Autodesk Fusion 360 part; units mm, degrees
note: some values were not read from the file. Set by a fixed rule: which sketch regions a step uses.
(part 10 of 20)
  spline S55 degree 5 poles (-13.208, 9.0304) (-13.2069, 9.0286) (-13.2047, 9.0249) (-13.2015, 9.0195) (-13.1971, 9.0122) (-13.1916, 9.0031) (-13.1862, 8.9941) (-13.1807, 8.9851) (-13.1752, 8.9761) (-13.1698, 8.9671) (-13.1643, 8.9582) (-13.1589, 8.9493) (-13.1534, 8.9405) (-13.1479, 8.9317) (-13.1425, 8.9229) (-13.137, 8.9141) (-13.1315, 8.9054) (-13.1261, 8.8967) (-13.1206, 8.888) (-13.1151, 8.8794) (-13.1097, 8.8708) (-13.1042, 8.8622) (-13.0988, 8.8537) (-13.0933, 8.8452) (-13.0878, 8.8367) (-13.0824, 8.8283) (-13.0769, 8.8199) (-13.0715, 8.8115) (-13.066, 8.8032) (-13.0606, 8.7948) (-13.0551, 8.7866) (-13.0497, 8.7783) (-13.0442, 8.7701) (-13.0388, 8.7619) (-13.0333, 8.7538) (-13.0279, 8.7456) (-13.0224, 8.7376) (-13.017, 8.7295) (-13.0116, 8.7215) (-13.0062, 8.7135) (-13.0007, 8.7055) (-12.9953, 8.6976) (-12.9899, 8.6897) (-12.9845, 8.6819) (-12.9791, 8.6741) (-12.9736, 8.6663) (-12.9682, 8.6585) (-12.9628, 8.6508) (-12.9574, 8.6431) (-12.9521, 8.6354) (-12.9467, 8.6278) (-12.9413, 8.6202) (-12.9359, 8.6126) (-12.9305, 8.6051) (-12.9252, 8.5976) (-12.9198, 8.5902) (-12.9144, 8.5827) (-12.9091, 8.5754) (-12.9037, 8.568) (-12.8984, 8.5607) (-12.893, 8.5534) (-12.8877, 8.5461) (-12.8824, 8.5389) (-12.8771, 8.5317) (-12.8718, 8.5246) (-12.8664, 8.5174) (-12.8611, 8.5103) (-12.8558, 8.5033) (-12.8506, 8.4963) (-12.8453, 8.4893) (-12.84, 8.4823) (-12.8347, 8.4754) (-12.8295, 8.4685) (-12.8242, 8.4617) (-12.819, 8.4549) (-12.8138, 8.4481) (-12.8085, 8.4413) (-12.8033, 8.4346) (-12.7981, 8.4279) (-12.7929, 8.4213) (-12.7877, 8.4147) (-12.7825, 8.4081) (-12.7773, 8.4016) (-12.7722, 8.3951) (-12.767, 8.3886) (-12.7619, 8.3822) (-12.7567, 8.3758) (-12.7516, 8.3694) (-12.7465, 8.3631) (-12.7414, 8.3568) (-12.7363, 8.3505) (-12.7312, 8.3443) (-12.7261, 8.3381) (-12.721, 8.332) (-12.716, 8.3259) (-12.7109, 8.3198) (-12.7059, 8.3137) (-12.7009, 8.3077) (-12.6959, 8.3017) (-12.6909, 8.2958) (-12.6859, 8.2899) (-12.6809, 8.284) (-12.676, 8.2782) (-12.671, 8.2724) (-12.6661, 8.2666) (-12.6612, 8.2609) (-12.6562, 8.2552) (-12.6513, 8.2496) (-12.6465, 8.2439) (-12.6416, 8.2384) (-12.6367, 8.2328) (-12.6319, 8.2273) (-12.6271, 8.2218) (-12.6223, 8.2164) (-12.6175, 8.211) (-12.6127, 8.2056) (-12.6079, 8.2003) (-12.6032, 8.195) (-12.5984, 8.1898) (-12.5937, 8.1846) (-12.589, 8.1794) (-12.5843, 8.1742) (-12.5796, 8.1691) (-12.575, 8.1641) (-12.5703, 8.159) (-12.5657, 8.154) (-12.5611, 8.1491) (-12.5565, 8.1441) (-12.552, 8.1393) (-12.5474, 8.1344) (-12.5429, 8.1296) (-12.5384, 8.1248) (-12.5339, 8.1201) (-12.5294, 8.1154) (-12.5249, 8.1107) (-12.5205, 8.1061) (-12.5161, 8.1015) (-12.5117, 8.097) (-12.5073, 8.0925) (-12.5029, 8.088) (-12.4986, 8.0836) (-12.4943, 8.0792) (-12.49, 8.0748) (-12.4857, 8.0705) (-12.4815, 8.0662) (-12.4772, 8.062) (-12.473, 8.0578) (-12.4688, 8.0536) (-12.4647, 8.0495) (-12.4605, 8.0454) (-12.4564, 8.0413) (-12.4523, 8.0373) (-12.4482, 8.0333) (-12.4442, 8.0294) (-12.4401, 8.0255) (-12.4361, 8.0216) (-12.4322, 8.0178) (-12.4282, 8.014) (-12.4243, 8.0103) (-12.4204, 8.0066) (-12.4165, 8.0029) (-12.4127, 7.9993) (-12.4089, 7.9957) (-12.4051, 7.9922) (-12.4013, 7.9887) (-12.3976, 7.9852) (-12.3938, 7.9818) (-12.3902, 7.9784) (-12.3865, 7.975) (-12.3829, 7.9717) (-12.3793, 7.9684) (-12.3757, 7.9652) (-12.3722, 7.962) (-12.3687, 7.9589) (-12.3652, 7.9558) (-12.3617, 7.9527) (-12.3583, 7.9496) (-12.3549, 7.9467) (-12.3516, 7.9437) (-12.3483, 7.9408) (-12.345, 7.9379) (-12.3417, 7.9351) (-12.3385, 7.9323) (-12.3353, 7.9296) (-12.3322, 7.9268) (-12.329, 7.9242) (-12.326, 7.9216) (-12.3229, 7.919) (-12.3199, 7.9164) (-12.3169, 7.9139) (-12.314, 7.9115) (-12.3111, 7.909) (-12.3082, 7.9066) (-12.3054, 7.9043) (-12.3026, 7.902) (-12.2998, 7.8998) (-12.2971, 7.8975) (-12.2944, 7.8954) (-12.2918, 7.8932) (-12.2892, 7.8911) (-12.2867, 7.8891) (-12.2841, 7.8871) (-12.2817, 7.8851) (-12.2792, 7.8832) (-12.2769, 7.8813) (-12.2745, 7.8795) (-12.2722, 7.8777) (-12.27, 7.8759) (-12.2677, 7.8742) (-12.2656, 7.8726) (-12.2635, 7.8709) (-12.2614, 7.8693) (-12.2594, 7.8678) (-12.2574, 7.8663) (-12.2555, 7.8649) (-12.2536, 7.8634) (-12.2517, 7.8621) (-12.25, 7.8608) (-12.2482, 7.8595) (-12.2465, 7.8582) (-12.2449, 7.857) (-12.2433, 7.8559) (-12.2418, 7.8548) (-12.2403, 7.8537) (-12.2389, 7.8527) (-12.2376, 7.8517) (-12.2363, 7.8508) (-12.235, 7.8499) (-12.2338, 7.8491) (-12.2327, 7.8483) (-12.2316, 7.8475) (-12.2306, 7.8468) (-12.2296, 7.8462) (-12.2287, 7.8455) (-12.2279, 7.845) (-12.2271, 7.8445) (-12.2264, 7.844) (-12.2258, 7.8435) (-12.2252, 7.8431) (-12.2247, 7.8428) (-12.2242, 7.8425) (-12.2239, 7.8423) (-12.2237, 7.8422) (-12.2236, 7.8421) (-12.2236, 7.8421) knots -1 -1 -1 -1 -1 -1 -0.99583333 -0.99166667 -0.9875 -0.98333333 -0.97916667 -0.975 -0.97083333 -0.96666667 -0.9625 -0.95833333 -0.95416667 -0.95 -0.94583333 -0.94166667 -0.9375 -0.93333333 -0.92916667 -0.925 -0.92083333 -0.91666667 -0.9125 -0.90833333 -0.90416667 -0.9 -0.89583333 -0.89166667 -0.8875 -0.88333333 -0.87916667 -0.875 -0.87083333 -0.86666667 -0.8625 -0.85833333 -0.85416667 -0.85 -0.84583333 -0.84166667 -0.8375 -0.83333333 -0.82916667 -0.825 -0.82083333 -0.81666667 -0.8125 -0.80833333 -0.80416667 -0.8 -0.79583333 -0.79166667 -0.7875 -0.78333333 -0.77916667 -0.775 -0.77083333 -0.76666667 -0.7625 -0.75833333 -0.75416667 -0.75 -0.74583333 -0.74166667 -0.7375 -0.73333333 -0.72916667 -0.725 -0.72083333 -0.71666667 -0.7125 -0.70833333 -0.70416667 -0.7 -0.69583333 -0.69166667 -0.6875 -0.68333333 -0.67916667 -0.675 -0.67083333 -0.66666667 -0.6625 -0.65833333 -0.65416667 -0.65 -0.64583333 -0.64166667 -0.6375 -0.63333333 -0.62916667 -0.625 -0.62083333 -0.61666667 -0.6125 -0.60833333 -0.60416667 -0.6 -0.59583333 -0.59166667 -0.5875 -0.58333333 -0.57916667 -0.575 -0.57083333 -0.56666667 -0.5625 -0.55833333 -0.55416667 -0.55 -0.54583333 -0.54166667 -0.5375 -0.53333333 -0.52916667 -0.525 -0.52083333 -0.51666667 -0.5125 -0.50833333 -0.50416667 -0.5 -0.49583333 -0.49166667 -0.4875 -0.48333333 -0.47916667 -0.475 -0.47083333 -0.46666667 -0.4625 -0.45833333 -0.45416667 -0.45 -0.44583333 -0.44166667 -0.4375 -0.43333333 -0.42916667 -0.425 -0.42083333 -0.41666667 -0.4125 -0.40833333 -0.40416667 -0.4 -0.39583333 -0.39166667 -0.3875 -0.38333333 -0.37916667 -0.375 -0.37083333 -0.36666667 -0.3625 -0.35833333 -0.35416667 -0.35 -0.34583333 -0.34166667 -0.3375 -0.33333333 -0.32916667 -0.325 -0.32083333 -0.31666667 -0.3125 -0.30833333 -0.30416667 -0.3 -0.29583333 -0.29166667 -0.2875 -0.28333333 -0.27916667 -0.275 -0.27083333 -0.26666667 -0.2625 -0.25833333 -0.25416667 -0.25 -0.24583333 -0.24166667 -0.2375 -0.23333333 -0.22916667 -0.225 -0.22083333 -0.21666667 -0.2125 -0.20833333 -0.20416667 -0.2 -0.19583333 -0.19166667 -0.1875 -0.18333333 -0.17916667 -0.175 -0.17083333 -0.16666667 -0.1625 -0.15833333 -0.15416667 -0.15 -0.14583333 -0.14166667 -0.1375 -0.13333333 -0.12916667 -0.125 -0.12083333 -0.11666667 -0.1125 -0.10833333 -0.10416667 -0.1 -0.09583333 -0.09166667 -0.0875 -0.08333333 -0.07916667 -0.075 -0.07083333 -0.06666667 -0.0625 -0.05833333 -0.05416667 -0.05 -0.04583333 -0.04166667 -0.0375 -0.03333333 -0.02916667 -0.025 -0.02083333 -0.01666667 -0.0125 -0.00833333 -0.00416667 0 0 0 0 0 0
  line L110 (-12.2236, 7.8421) -> (-12.223, 7.8417)
  line L111 (-12.223, 7.8417) -> (-11.5731, 7.4247)
  arc A56 (-11.5731, 7.4247) -> (-12.2165, 6.3102) centre (0, 0) ccw
  line L112 (-12.2165, 6.3102) -> (-12.9026, 6.6646)
  line L113 (-12.9026, 6.6646) -> (-12.9032, 6.6649)
  spline S56 degree 5 poles (-12.9032, 6.6649) (-12.9033, 6.6649) (-12.9034, 6.665) (-12.9036, 6.6651) (-12.9039, 6.6652) (-12.9044, 6.6655) (-12.905, 6.6658) (-12.9056, 6.6661) (-12.9063, 6.6664) (-12.9071, 6.6668) (-12.9079, 6.6672) (-12.9088, 6.6676) (-12.9098, 6.6681) (-12.9108, 6.6686) (-12.912, 6.6691) (-12.9132, 6.6697) (-12.9144, 6.6703) (-12.9157, 6.6709) (-12.9171, 6.6715) (-12.9186, 6.6722) (-12.9201, 6.6729) (-12.9217, 6.6736) (-12.9234, 6.6743) (-12.9251, 6.6751) (-12.9269, 6.6759) (-12.9287, 6.6767) (-12.9306, 6.6775) (-12.9326, 6.6784) (-12.9346, 6.6793) (-12.9367, 6.6802) (-12.9389, 6.6811) (-12.9411, 6.6821) (-12.9434, 6.683) (-12.9457, 6.684) (-12.9482, 6.685) (-12.9506, 6.686) (-12.9531, 6.6871) (-12.9557, 6.6881) (-12.9584, 6.6892) (-12.9611, 6.6903) (-12.9638, 6.6914) (-12.9667, 6.6925) (-12.9695, 6.6937) (-12.9725, 6.6948) (-12.9755, 6.696) (-12.9785, 6.6972) (-12.9816, 6.6984) (-12.9848, 6.6996) (-12.988, 6.7008) (-12.9913, 6.7021) (-12.9946, 6.7033) (-12.998, 6.7046) (-13.0015, 6.7059) (-13.005, 6.7072) (-13.0085, 6.7085) (-13.0121, 6.7098) (-13.0158, 6.7111) (-13.0195, 6.7125) (-13.0232, 6.7138) (-13.0271, 6.7152) (-13.0309, 6.7165) (-13.0349, 6.7179) (-13.0388, 6.7193) (-13.0429, 6.7207) (-13.0469, 6.7221) (-13.0511, 6.7235) (-13.0552, 6.7249) (-13.0595, 6.7264) (-13.0638, 6.7278) (-13.0681, 6.7292) (-13.0725, 6.7307) (-13.0769, 6.7321) (-13.0814, 6.7336) (-13.0859, 6.7351) (-13.0905, 6.7366) (-13.0951, 6.738) (-13.0998, 6.7395) (-13.1046, 6.741) (-13.1093, 6.7425) (-13.1142, 6.744) (-13.119, 6.7455) (-13.124, 6.747) (-13.1289, 6.7485) (-13.1339, 6.75) (-13.139, 6.7516) (-13.1441, 6.7531) (-13.1493, 6.7546) (-13.1545, 6.7561) (-13.1597, 6.7577) (-13.165, 6.7592) (-13.1704, 6.7607) (-13.1758, 6.7623) (-13.1812, 6.7638) (-13.1867, 6.7653) (-13.1922, 6.7669) (-13.1978, 6.7684) (-13.2034, 6.77) (-13.209, 6.7715) (-13.2147, 6.7731) (-13.2205, 6.7746) (-13.2263, 6.7761) (-13.2321, 6.7777) (-13.238, 6.7792) (-13.2439, 6.7808) (-13.2499, 6.7823) (-13.2559, 6.7839) (-13.2619, 6.7854) (-13.268, 6.7869) (-13.2742, 6.7885) (-13.2804, 6.79) (-13.2866, 6.7915) (-13.2928, 6.7931) (-13.2991, 6.7946) (-13.3055, 6.7961) (-13.3119, 6.7976) (-13.3183, 6.7992) (-13.3248, 6.8007) (-13.3313, 6.8022) (-13.3379, 6.8037) (-13.3445, 6.8052) (-13.3511, 6.8067) (-13.3578, 6.8082) (-13.3645, 6.8097) (-13.3712, 6.8112) (-13.378, 6.8127) (-13.3849, 6.8142) (-13.3918, 6.8157) (-13.3987, 6.8171) (-13.4056, 6.8186) (-13.4126, 6.8201) (-13.4197, 6.8215) (-13.4267, 6.823) (-13.4339, 6.8244) (-13.441, 6.8259) (-13.4482, 6.8273) (-13.4554, 6.8288) (-13.4627, 6.8302) (-13.47, 6.8316) (-13.4773, 6.833) (-13.4847, 6.8344) (-13.4922, 6.8358) (-13.4996, 6.8372) (-13.5071, 6.8386) (-13.5146, 6.84) (-13.5222, 6.8414) (-13.5298, 6.8427) (-13.5375, 6.8441) (-13.5451, 6.8454) (-13.5528, 6.8468) (-13.5606, 6.8481) (-13.5684, 6.8494) (-13.5762, 6.8508) (-13.5841, 6.8521) (-13.592, 6.8534) (-13.5999, 6.8547) (-13.6079, 6.856) (-13.6159, 6.8572) (-13.6239, 6.8585) (-13.632, 6.8598) (-13.6401, 6.861) (-13.6483, 6.8623) (-13.6564, 6.8635) (-13.6647, 6.8647) (-13.6729, 6.8659) (-13.6812, 6.8671) (-13.6895, 6.8683) (-13.6979, 6.8695) (-13.7063, 6.8707) (-13.7147, 6.8718) (-13.7231, 6.873) (-13.7316, 6.8741) (-13.7401, 6.8753) (-13.7487, 6.8764) (-13.7573, 6.8775) (-13.7659, 6.8786) (-13.7746, 6.8797) (-13.7833, 6.8808) (-13.792, 6.8818) (-13.8007, 6.8829) (-13.8095, 6.884) (-13.8184, 6.885) (-13.8272, 6.886) (-13.8361, 6.887) (-13.845, 6.888) (-13.854, 6.889) (-13.8629, 6.89) (-13.872, 6.891) (-13.881, 6.8919) (-13.8901, 6.8929) (-13.8992, 6.8938) (-13.9083, 6.8947) (-13.9175, 6.8956) (-13.9267, 6.8965) (-13.936, 6.8974) (-13.9452, 6.8982) (-13.9545, 6.8991) (-13.9639, 6.8999) (-13.9732, 6.9008) (-13.9826, 6.9016) (-13.992, 6.9024) (-14.0015, 6.9032) (-14.011, 6.9039) (-14.0205, 6.9047) (-14.03, 6.9055) (-14.0396, 6.9062) (-14.0492, 6.9069) (-14.0588, 6.9076) (-14.0685, 6.9083) (-14.0782, 6.909) (-14.0879, 6.9097) (-14.0976, 6.9103) (-14.1074, 6.9109) (-14.1172, 6.9116) (-14.1271, 6.9122) (-14.1369, 6.9128) (-14.1468, 6.9134) (-14.1568, 6.9139) (-14.1667, 6.9145) (-14.1767, 6.915) (-14.1867, 6.9155) (-14.1967, 6.916) (-14.2068, 6.9165) (-14.2169, 6.917) (-14.227, 6.9175) (-14.2372, 6.9179) (-14.2474, 6.9183) (-14.2576, 6.9188) (-14.2678, 6.9192) (-14.2781, 6.9195) (-14.2883, 6.9199) (-14.2987, 6.9203) (-14.309, 6.9206) (-14.3194, 6.9209) (-14.3298, 6.9212) (-14.3402, 6.9215) (-14.3507, 6.9218) (-14.3611, 6.9221) (-14.3716, 6.9223) (-14.3822, 6.9225) (-14.3927, 6.9227) (-14.4033, 6.9229) (-14.4118, 6.9231) (-14.4182, 6.9232) (-14.4224, 6.9232) (-14.4246, 6.9233) knots 0 0 0 0 0 0 0.00416667 0.00833333 0.0125 0.01666667 0.02083333 0.025 0.02916667 0.03333333 0.0375 0.04166667 0.04583333 0.05 0.05416667 0.05833333 0.0625 0.06666667 0.07083333 0.075 0.07916667 0.08333333 0.0875 0.09166667 0.09583333 0.1 0.10416667 0.10833333 0.1125 0.11666667 0.12083333 0.125 0.12916667 0.13333333 0.1375 0.14166667 0.14583333 0.15 0.15416667 0.15833333 0.1625 0.16666667 0.17083333 0.175 0.17916667 0.18333333 0.1875 0.19166667 0.19583333 0.2 0.20416667 0.20833333 0.2125 0.21666667 0.22083333 0.225 0.22916667 0.23333333 0.2375 0.24166667 0.24583333 0.25 0.25416667 0.25833333 0.2625 0.26666667 0.27083333 0.275 0.27916667 0.28333333 0.2875 0.29166667 0.29583333 0.3 0.30416667 0.30833333 0.3125 0.31666667 0.32083333 0.325 0.32916667 0.33333333 0.3375 0.34166667 0.34583333 0.35 0.35416667 0.35833333 0.3625 0.36666667 0.37083333 0.375 0.37916667 0.38333333 0.3875 0.39166667 0.39583333 0.4 0.40416667 0.40833333 0.4125 0.41666667 0.42083333 0.425 0.42916667 0.43333333 0.4375 0.44166667 0.44583333 0.45 0.45416667 0.45833333 0.4625 0.46666667 0.47083333 0.475 0.47916667 0.48333333 0.4875 0.49166667 0.49583333 0.5 0.50416667 0.50833333 0.5125 0.51666667 0.52083333 0.525 0.52916667 0.53333333 0.5375 0.54166667 0.54583333 0.55 0.55416667 0.55833333 0.5625 0.56666667 0.57083333 0.575 0.57916667 0.58333333 0.5875 0.59166667 0.59583333 0.6 0.60416667 0.60833333 0.6125 0.61666667 0.62083333 0.625 0.62916667 0.63333333 0.6375 0.64166667 0.64583333 0.65 0.65416667 0.65833333 0.6625 0.66666667 0.67083333 0.675 0.67916667 0.68333333 0.6875 0.69166667 0.69583333 0.7 0.70416667 0.70833333 0.7125 0.71666667 0.72083333 0.725 0.72916667 0.73333333 0.7375 0.74166667 0.74583333 0.75 0.75416667 0.75833333 0.7625 0.76666667 0.77083333 0.775 0.77916667 0.78333333 0.7875 0.79166667 0.79583333 0.8 0.80416667 0.80833333 0.8125 0.81666667 0.82083333 0.825 0.82916667 0.83333333 0.8375 0.84166667 0.84583333 0.85 0.85416667 0.85833333 0.8625 0.86666667 0.87083333 0.875 0.87916667 0.88333333 0.8875 0.89166667 0.89583333 0.9 0.90416667 0.90833333 0.9125 0.91666667 0.92083333 0.925 0.92916667 0.93333333 0.9375 0.94166667 0.94583333 0.95 0.95416667 0.95833333 0.9625 0.96666667 0.97083333 0.975 0.97916667 0.98333333 0.9875 0.99166667 0.99583333 1 1 1 1 1 1
  arc A57 (-14.4246, 6.9233) -> (-14.7969, 6.087) centre (0, 0) ccw
  spline S57 degree 5 poles (-14.7969, 6.087) (-14.7955, 6.0854) (-14.7926, 6.0823) (-14.7882, 6.0776) (-14.7824, 6.0714) (-14.7752, 6.0637) (-14.768, 6.056) (-14.7608, 6.0483) (-14.7536, 6.0406) (-14.7464, 6.033) (-14.7392, 6.0254) (-14.732, 6.0179) (-14.7248, 6.0104) (-14.7176, 6.0029) (-14.7104, 5.9954) (-14.7033, 5.988) (-14.6961, 5.9806) (-14.689, 5.9732) (-14.6818, 5.9659) (-14.6747, 5.9586) (-14.6675, 5.9513) (-14.6604, 5.9441) (-14.6533, 5.9368) (-14.6462, 5.9297) (-14.6391, 5.9225) (-14.632, 5.9154) (-14.6249, 5.9083) (-14.6178, 5.9012) (-14.6108, 5.8942) (-14.6037, 5.8872) (-14.5966, 5.8802) (-14.5896, 5.8733) (-14.5826, 5.8664) (-14.5755, 5.8595) (-14.5685, 5.8527) (-14.5615, 5.8459) (-14.5545, 5.8391) (-14.5475, 5.8324) (-14.5405, 5.8256) (-14.5336, 5.819) (-14.5266, 5.8123) (-14.5197, 5.8057) (-14.5127, 5.7991) (-14.5058, 5.7925) (-14.4989, 5.786) (-14.492, 5.7795) (-14.4851, 5.773) (-14.4782, 5.7666) (-14.4713, 5.7602) (-14.4644, 5.7538) (-14.4576, 5.7475) (-14.4507, 5.7412) (-14.4439, 5.7349) (-14.4371, 5.7287) (-14.4303, 5.7225) (-14.4235, 5.7163) (-14.4167, 5.7101) (-14.4099, 5.704) (-14.4031, 5.6979) (-14.3964, 5.6919) (-14.3896, 5.6859) (-14.3829, 5.6799) (-14.3762, 5.6739) (-14.3695, 5.668) (-14.3628, 5.6621) (-14.3562, 5.6562) (-14.3495, 5.6504) (-14.3429, 5.6446) (-14.3362, 5.6388) (-14.3296, 5.6331) (-14.323, 5.6274) (-14.3164, 5.6217) (-14.3098, 5.6161) (-14.3033, 5.6105) (-14.2967, 5.6049) (-14.2902, 5.5993) (-14.2837, 5.5938) (-14.2772, 5.5883) (-14.2707, 5.5829) (-14.2642, 5.5775) (-14.2578, 5.5721) (-14.2513, 5.5667) (-14.2449, 5.5614) (-14.2385, 5.5561) (-14.2321, 5.5509) (-14.2257, 5.5457) (-14.2194, 5.5405) (-14.213, 5.5353) (-14.2067, 5.5302) (-14.2004, 5.5251) (-14.1941, 5.52) (-14.1879, 5.515) (-14.1816, 5.51) (-14.1754, 5.505) (-14.1692, 5.5001) (-14.163, 5.4952) (-14.1568, 5.4903) (-14.1506, 5.4855) (-14.1445, 5.4807) (-14.1383, 5.4759) (-14.1322, 5.4712) (-14.1262, 5.4665) (-14.1201, 5.4618) (-14.114, 5.4572) (-14.108, 5.4526) (-14.102, 5.448) (-14.096, 5.4434) (-14.0901, 5.4389) (-14.0841, 5.4344) (-14.0782, 5.43) (-14.0723, 5.4256) (-14.0664, 5.4212) (-14.0606, 5.4169) (-14.0547, 5.4125) (-14.0489, 5.4083) (-14.0431, 5.404) (-14.0373, 5.3998) (-14.0316, 5.3956) (-14.0259, 5.3914) (-14.0202, 5.3873) (-14.0145, 5.3832) (-14.0088, 5.3792) (-14.0032, 5.3752) (-13.9976, 5.3712) (-13.992, 5.3672) (-13.9865, 5.3633) (-13.9809, 5.3594) (-13.9754, 5.3555) (-13.9699, 5.3517) (-13.9645, 5.3479) (-13.959, 5.3441) (-13.9536, 5.3404) (-13.9482, 5.3367) (-13.9429, 5.3331) (-13.9376, 5.3294) (-13.9322, 5.3258) (-13.927, 5.3223) (-13.9217, 5.3187) (-13.9165, 5.3152) (-13.9113, 5.3118) (-13.9061, 5.3083) (-13.901, 5.3049) (-13.8959, 5.3015) (-13.8908, 5.2982) (-13.8858, 5.2949) (-13.8807, 5.2916) (-13.8757, 5.2884) (-13.8708, 5.2852) (-13.8658, 5.282) (-13.8609, 5.2789) (-13.8561, 5.2758) (-13.8512, 5.2727) (-13.8464, 5.2697) (-13.8416, 5.2666) (-13.8369, 5.2637) (-13.8322, 5.2607) (-13.8275, 5.2578) (-13.8228, 5.2549) (-13.8182, 5.2521) (-13.8136, 5.2493) (-13.8091, 5.2465) (-13.8046, 5.2438) (-13.8001, 5.241) (-13.7956, 5.2384) (-13.7912, 5.2357) (-13.7869, 5.2331) (-13.7825, 5.2305) (-13.7782, 5.228) (-13.7739, 5.2254) (-13.7697, 5.223) (-13.7655, 5.2205) (-13.7613, 5.2181) (-13.7572, 5.2157) (-13.7531, 5.2134) (-13.7491, 5.211) (-13.7451, 5.2087) (-13.7411, 5.2065) (-13.7372, 5.2043) (-13.7333, 5.2021) (-13.7294, 5.1999) (-13.7256, 5.1978) (-13.7218, 5.1957) (-13.7181, 5.1936) (-13.7144, 5.1916) (-13.7108, 5.1896) (-13.7072, 5.1877) (-13.7036, 5.1857) (-13.7001, 5.1838) (-13.6966, 5.182) (-13.6932, 5.1801) (-13.6898, 5.1783) (-13.6864, 5.1766) (-13.6831, 5.1749) (-13.6799, 5.1732) (-13.6767, 5.1715) (-13.6735, 5.1698) (-13.6704, 5.1682) (-13.6673, 5.1667) (-13.6643, 5.1651) (-13.6613, 5.1636) (-13.6584, 5.1622) (-13.6555, 5.1607) (-13.6527, 5.1593) (-13.6499, 5.1579) (-13.6472, 5.1566) (-13.6445, 5.1553) (-13.6419, 5.154) (-13.6393, 5.1528) (-13.6368, 5.1515) (-13.6343, 5.1504) (-13.6319, 5.1492) (-13.6296, 5.1481) (-13.6273, 5.147) (-13.625, 5.146) (-13.6228, 5.1449) (-13.6207, 5.1439) (-13.6186, 5.143) (-13.6166, 5.1421) (-13.6147, 5.1412) (-13.6128, 5.1403) (-13.6109, 5.1395) (-13.6091, 5.1387) (-13.6074, 5.1379) (-13.6057, 5.1372) (-13.6042, 5.1365) (-13.6026, 5.1358) (-13.6011, 5.1352) (-13.5997, 5.1346) (-13.5984, 5.134) (-13.5971, 5.1335) (-13.5959, 5.1329) (-13.5948, 5.1325) (-13.5937, 5.132) (-13.5927, 5.1316) (-13.5918, 5.1312) (-13.5909, 5.1309) (-13.5901, 5.1305) (-13.5894, 5.1303) (-13.5887, 5.13) (-13.5882, 5.1298) (-13.5877, 5.1296) (-13.5873, 5.1294) (-13.5871, 5.1293) (-13.587, 5.1293) (-13.5869, 5.1293) knots -1 -1 -1 -1 -1 -1 -0.99583333 -0.99166667 -0.9875 -0.98333333 -0.97916667 -0.975 -0.97083333 -0.96666667 -0.9625 -0.95833333 -0.95416667 -0.95 -0.94583333 -0.94166667 -0.9375 -0.93333333 -0.92916667 -0.925 -0.92083333 -0.91666667 -0.9125 -0.90833333 -0.90416667 -0.9 -0.89583333 -0.89166667 -0.8875 -0.88333333 -0.87916667 -0.875 -0.87083333 -0.86666667 -0.8625 -0.85833333 -0.85416667 -0.85 -0.84583333 -0.84166667 -0.8375 -0.83333333 -0.82916667 -0.825 -0.82083333 -0.81666667 -0.8125 -0.80833333 -0.80416667 -0.8 -0.79583333 -0.79166667 -0.7875 -0.78333333 -0.77916667 -0.775 -0.77083333 -0.76666667 -0.7625 -0.75833333 -0.75416667 -0.75 -0.74583333 -0.74166667 -0.7375 -0.73333333 -0.72916667 -0.725 -0.72083333 -0.71666667 -0.7125 -0.70833333 -0.70416667 -0.7 -0.69583333 -0.69166667 -0.6875 -0.68333333 -0.67916667 -0.675 -0.67083333 -0.66666667 -0.6625 -0.65833333 -0.65416667 -0.65 -0.64583333 -0.64166667 -0.6375 -0.63333333 -0.62916667 -0.625 -0.62083333 -0.61666667 -0.6125 -0.60833333 -0.60416667 -0.6 -0.59583333 -0.59166667 -0.5875 -0.58333333 -0.57916667 -0.575 -0.57083333 -0.56666667 -0.5625 -0.55833333 -0.55416667 -0.55 -0.54583333 -0.54166667 -0.5375 -0.53333333 -0.52916667 -0.525 -0.52083333 -0.51666667 -0.5125 -0.50833333 -0.50416667 -0.5 -0.49583333 -0.49166667 -0.4875 -0.48333333 -0.47916667 -0.475 -0.47083333 -0.46666667 -0.4625 -0.45833333 -0.45416667 -0.45 -0.44583333 -0.44166667 -0.4375 -0.43333333 -0.42916667 -0.425 -0.42083333 -0.41666667 -0.4125 -0.40833333 -0.40416667 -0.4 -0.39583333 -0.39166667 -0.3875 -0.38333333 -0.37916667 -0.375 -0.37083333 -0.36666667 -0.3625 -0.35833333 -0.35416667 -0.35 -0.34583333 -0.34166667 -0.3375 -0.33333333 -0.32916667 -0.325 -0.32083333 -0.31666667 -0.3125 -0.30833333 -0.30416667 -0.3 -0.29583333 -0.29166667 -0.2875 -0.28333333 -0.27916667 -0.275 -0.27083333 -0.26666667 -0.2625 -0.25833333 -0.25416667 -0.25 -0.24583333 -0.24166667 -0.2375 -0.23333333 -0.22916667 -0.225 -0.22083333 -0.21666667 -0.2125 -0.20833333 -0.20416667 -0.2 -0.19583333 -0.19166667 -0.1875 -0.18333333 -0.17916667 -0.175 -0.17083333 -0.16666667 -0.1625 -0.15833333 -0.15416667 -0.15 -0.14583333 -0.14166667 -0.1375 -0.13333333 -0.12916667 -0.125 -0.12083333 -0.11666667 -0.1125 -0.10833333 -0.10416667 -0.1 -0.09583333 -0.09166667 -0.0875 -0.08333333 -0.07916667 -0.075 -0.07083333 -0.06666667 -0.0625 -0.05833333 -0.05416667 -0.05 -0.04583333 -0.04166667 -0.0375 -0.03333333 -0.02916667 -0.025 -0.02083333 -0.01666667 -0.0125 -0.00833333 -0.00416667 0 0 0 0 0 0
  line L114 (-13.5869, 5.1293) -> (-13.5863, 5.129)
  line L115 (-13.5863, 5.129) -> (-12.8639, 4.8563)
  arc A58 (-12.8639, 4.8563) -> (-13.2615, 3.6324) centre (0, 0) ccw
  line L116 (-13.2615, 3.6324) -> (-14.0063, 3.8363)
  line L117 (-14.0063, 3.8363) -> (-14.007, 3.8365)
  spline S58 degree 5 poles (-14.007, 3.8365) (-14.007, 3.8365) (-14.0072, 3.8366) (-14.0074, 3.8366) (-14.0077, 3.8367) (-14.0083, 3.8369) (-14.0089, 3.837) (-14.0095, 3.8372) (-14.0103, 3.8374) (-14.0111, 3.8376) (-14.012, 3.8378) (-14.013, 3.838) (-14.0141, 3.8383) (-14.0152, 3.8386) (-14.0164, 3.8388) (-14.0177, 3.8391) (-14.019, 3.8394) (-14.0204, 3.8398) (-14.0219, 3.8401) (-14.0235, 3.8405) (-14.0251, 3.8408) (-14.0268, 3.8412) (-14.0286, 3.8416) (-14.0305, 3.842) (-14.0324, 3.8424) (-14.0343, 3.8428) (-14.0364, 3.8432) (-14.0385, 3.8436) (-14.0407, 3.8441) (-14.0429, 3.8445) (-14.0452, 3.845) (-14.0476, 3.8454) (-14.05, 3.8459) (-14.0525, 3.8464) (-14.0551, 3.8469) (-14.0577, 3.8473) (-14.0604, 3.8478) (-14.0632, 3.8483) (-14.066, 3.8488) (-14.0688, 3.8493) (-14.0718, 3.8498) (-14.0748, 3.8504) (-14.0778, 3.8509) (-14.0809, 3.8514) (-14.0841, 3.8519) (-14.0873, 3.8525) (-14.0906, 3.853) (-14.094, 3.8535) (-14.0974, 3.854) (-14.1009, 3.8546) (-14.1044, 3.8551) (-14.1079, 3.8557) (-14.1116, 3.8562) (-14.1153, 3.8567) (-14.119, 3.8573) (-14.1228, 3.8578) (-14.1267, 3.8583) (-14.1306, 3.8589) (-14.1345, 3.8594) (-14.1386, 3.86) (-14.1426, 3.8605) (-14.1467, 3.861) (-14.1509, 3.8615) (-14.1552, 3.8621) (-14.1594, 3.8626) (-14.1638, 3.8631) (-14.1682, 3.8636) (-14.1726, 3.8642) (-14.1771, 3.8647) (-14.1816, 3.8652) (-14.1862, 3.8657) (-14.1908, 3.8662) (-14.1955, 3.8667) (-14.2003, 3.8672) (-14.2051, 3.8677) (-14.2099, 3.8682) (-14.2148, 3.8686) (-14.2197, 3.8691) (-14.2247, 3.8696) (-14.2297, 3.87) (-14.2348, 3.8705) (-14.2399, 3.871) (-14.2451, 3.8714) (-14.2503, 3.8718) (-14.2556, 3.8723) (-14.2609, 3.8727) (-14.2663, 3.8731) (-14.2717, 3.8735) (-14.2771, 3.8739) (-14.2826, 3.8743) (-14.2882, 3.8747) (-14.2938, 3.8751) (-14.2994, 3.8755) (-14.3051, 3.8758) (-14.3108, 3.8762) (-14.3166, 3.8766) (-14.3224, 3.8769) (-14.3283, 3.8772) (-14.3342, 3.8776) (-14.3401, 3.8779) (-14.3461, 3.8782) (-14.3521, 3.8785) (-14.3582, 3.8788) (-14.3643, 3.879) (-14.3705, 3.8793) (-14.3767, 3.8796) (-14.3829, 3.8798) (-14.3892, 3.88) (-14.3955, 3.8803) (-14.4019, 3.8805) (-14.4083, 3.8807) (-14.4147, 3.8809) (-14.4212, 3.8811) (-14.4277, 3.8812) (-14.4343, 3.8814) (-14.4409, 3.8816) (-14.4476, 3.8817) (-14.4542, 3.8818) (-14.461, 3.8819) (-14.4677, 3.882) (-14.4745, 3.8821) (-14.4814, 3.8822) (-14.4883, 3.8823) (-14.4952, 3.8823) (-14.5021, 3.8824) (-14.5091, 3.8824) (-14.5162, 3.8824) (-14.5233, 3.8824) (-14.5304, 3.8824) (-14.5375, 3.8824) (-14.5447, 3.8824) (-14.5519, 3.8823) (-14.5592, 3.8823) (-14.5665, 3.8822) (-14.5738, 3.8821) (-14.5812, 3.882) (-14.5886, 3.8819) (-14.596, 3.8817) (-14.6035, 3.8816) (-14.611, 3.8814) (-14.6186, 3.8813) (-14.6261, 3.8811) (-14.6338, 3.8809) (-14.6414, 3.8807) (-14.6491, 3.8804) (-14.6568, 3.8802) (-14.6646, 3.8799) (-14.6724, 3.8797) (-14.6802, 3.8794) (-14.6881, 3.8791) (-14.696, 3.8787) (-14.7039, 3.8784) (-14.7119, 3.878) (-14.7199, 3.8777) (-14.7279, 3.8773) (-14.7359, 3.8769) (-14.744, 3.8765) (-14.7522, 3.8761) (-14.7603, 3.8756) (-14.7685, 3.8751) (-14.7768, 3.8747) (-14.785, 3.8742) (-14.7933, 3.8737) (-14.8016, 3.8731) (-14.81, 3.8726) (-14.8184, 3.872) (-14.8268, 3.8714) (-14.8352, 3.8708) (-14.8437, 3.8702) (-14.8522, 3.8696) (-14.8608, 3.869) (-14.8693, 3.8683) (-14.8779, 3.8676) (-14.8866, 3.8669) (-14.8952, 3.8662) (-14.9039, 3.8655) (-14.9127, 3.8647) (-14.9214, 3.8639) (-14.9302, 3.8632) (-14.939, 3.8624) (-14.9479, 3.8615) (-14.9567, 3.8607) (-14.9656, 3.8598) (-14.9746, 3.859) (-14.9835, 3.8581) (-14.9925, 3.8572) (-15.0015, 3.8562) (-15.0106, 3.8553) (-15.0197, 3.8543) (-15.0288, 3.8533) (-15.0379, 3.8523) (-15.0471, 3.8513) (-15.0563, 3.8503) (-15.0655, 3.8492) (-15.0747, 3.8481) (-15.084, 3.847) (-15.0933, 3.8459) (-15.1026, 3.8448) (-15.112, 3.8436) (-15.1214, 3.8424) (-15.1308, 3.8412) (-15.1402, 3.84) (-15.1497, 3.8388) (-15.1591, 3.8375) (-15.1687, 3.8363) (-15.1782, 3.835) (-15.1878, 3.8337) (-15.1974, 3.8323) (-15.207, 3.831) (-15.2166, 3.8296) (-15.2263, 3.8282) (-15.236, 3.8268) (-15.2457, 3.8254) (-15.2555, 3.8239) (-15.2653, 3.8225) (-15.2751, 3.821) (-15.2849, 3.8195) (-15.2947, 3.8179) (-15.3046, 3.8164) (-15.3145, 3.8148) (-15.3244, 3.8132) (-15.3344, 3.8116) (-15.3444, 3.81) (-15.3544, 3.8083) (-15.3644, 3.8067) (-15.3744, 3.805) (-15.3845, 3.8033) (-15.3946, 3.8015) (-15.4047, 3.7998) (-15.4148, 3.798) (-15.425, 3.7962) (-15.4352, 3.7944) (-15.4454, 3.7925) (-15.4556, 3.7907) (-15.4659, 3.7888) (-15.4762, 3.7869) (-15.4865, 3.7849) (-15.4968, 3.783) (-15.5072, 3.781) (-15.5175, 3.779) (-15.5279, 3.777) (-15.5363, 3.7754) (-15.5425, 3.7742) (-15.5467, 3.7733) (-15.5488, 3.7729) knots 0 0 0 0 0 0 0.00416667 0.00833333 0.0125 0.01666667 0.02083333 0.025 0.02916667 0.03333333 0.0375 0.04166667 0.04583333 0.05 0.05416667 0.05833333 0.0625 0.06666667 0.07083333 0.075 0.07916667 0.08333333 0.0875 0.09166667 0.09583333 0.1 0.10416667 0.10833333 0.1125 0.11666667 0.12083333 0.125 0.12916667 0.13333333 0.1375 0.14166667 0.14583333 0.15 0.15416667 0.15833333 0.1625 0.16666667 0.17083333 0.175 0.17916667 0.18333333 0.1875 0.19166667 0.19583333 0.2 0.20416667 0.20833333 0.2125 0.21666667 0.22083333 0.225 0.22916667 0.23333333 0.2375 0.24166667 0.24583333 0.25 0.25416667 0.25833333 0.2625 0.26666667 0.27083333 0.275 0.27916667 0.28333333 0.2875 0.29166667 0.29583333 0.3 0.30416667 0.30833333 0.3125 0.31666667 0.32083333 0.325 0.32916667 0.33333333 0.3375 0.34166667 0.34583333 0.35 0.35416667 0.35833333 0.3625 0.36666667 0.37083333 0.375 0.37916667 0.38333333 0.3875 0.39166667 0.39583333 0.4 0.40416667 0.40833333 0.4125 0.41666667 0.42083333 0.425 0.42916667 0.43333333 0.4375 0.44166667 0.44583333 0.45 0.45416667 0.45833333 0.4625 0.46666667 0.47083333 0.475 0.47916667 0.48333333 0.4875 0.49166667 0.49583333 0.5 0.50416667 0.50833333 0.5125 0.51666667 0.52083333 0.525 0.52916667 0.53333333 0.5375 0.54166667 0.54583333 0.55 0.55416667 0.55833333 0.5625 0.56666667 0.57083333 0.575 0.57916667 0.58333333 0.5875 0.59166667 0.59583333 0.6 0.60416667 0.60833333 0.6125 0.61666667 0.62083333 0.625 0.62916667 0.63333333 0.6375 0.64166667 0.64583333 0.65 0.65416667 0.65833333 0.6625 0.66666667 0.67083333 0.675 0.67916667 0.68333333 0.6875 0.69166667 0.69583333 0.7 0.70416667 0.70833333 0.7125 0.71666667 0.72083333 0.725 0.72916667 0.73333333 0.7375 0.74166667 0.74583333 0.75 0.75416667 0.75833333 0.7625 0.76666667 0.77083333 0.775 0.77916667 0.78333333 0.7875 0.79166667 0.79583333 0.8 0.80416667 0.80833333 0.8125 0.81666667 0.82083333 0.825 0.82916667 0.83333333 0.8375 0.84166667 0.84583333 0.85 0.85416667 0.85833333 0.8625 0.86666667 0.87083333 0.875 0.87916667 0.88333333 0.8875 0.89166667 0.89583333 0.9 0.90416667 0.90833333 0.9125 0.91666667 0.92083333 0.925 0.92916667 0.93333333 0.9375 0.94166667 0.94583333 0.95 0.95416667 0.95833333 0.9625 0.96666667 0.97083333 0.975 0.97916667 0.98333333 0.9875 0.99166667 0.99583333 1 1 1 1 1 1
  arc A59 (-15.5488, 3.7729) -> (-15.7391, 2.8775) centre (0, 0) ccw
  spline S59 degree 5 poles (-15.7391, 2.8775) (-15.7374, 2.8763) (-15.7339, 2.8738) (-15.7287, 2.8702) (-15.7217, 2.8653) (-15.713, 2.8592) (-15.7044, 2.8532) (-15.6957, 2.8472) (-15.6871, 2.8412) (-15.6785, 2.8353) (-15.6698, 2.8293) (-15.6612, 2.8234) (-15.6526, 2.8176) (-15.6441, 2.8117) (-15.6355, 2.8059) (-15.6269, 2.8002) (-15.6184, 2.7944) (-15.6099, 2.7887) (-15.6014, 2.783) (-15.5929, 2.7773) (-15.5844, 2.7717) (-15.5759, 2.7661) (-15.5674, 2.7605) (-15.559, 2.755) (-15.5505, 2.7494) (-15.5421, 2.744) (-15.5337, 2.7385) (-15.5253, 2.7331) (-15.517, 2.7277) (-15.5086, 2.7223) (-15.5002, 2.7169) (-15.4919, 2.7116) (-15.4836, 2.7063) (-15.4753, 2.7011) (-15.467, 2.6958) (-15.4587, 2.6906) (-15.4505, 2.6855) (-15.4422, 2.6803) (-15.434, 2.6752) (-15.4258, 2.6701) (-15.4176, 2.665) (-15.4094, 2.66) (-15.4013, 2.655) (-15.3931, 2.65) (-15.385, 2.6451) (-15.3769, 2.6402) (-15.3688, 2.6353) (-15.3607, 2.6304) (-15.3527, 2.6256) (-15.3446, 2.6208) (-15.3366, 2.616) (-15.3286, 2.6113) (-15.3206, 2.6065) (-15.3126, 2.6019) (-15.3047, 2.5972) (-15.2968, 2.5926) (-15.2888, 2.588) (-15.2809, 2.5834) (-15.2731, 2.5788) (-15.2652, 2.5743) (-15.2574, 2.5698) (-15.2495, 2.5654) (-15.2417, 2.5609) (-15.2339, 2.5565) (-15.2262, 2.5522) (-15.2184, 2.5478) (-15.2107, 2.5435) (-15.203, 2.5392) (-15.1953, 2.5349) (-15.1876, 2.5307) (-15.18, 2.5265) (-15.1724, 2.5223) (-15.1648, 2.5182) (-15.1572, 2.514) (-15.1496, 2.5099) (-15.1421, 2.5059) (-15.1346, 2.5018) (-15.1271, 2.4978) (-15.1196, 2.4939) (-15.1121, 2.4899) (-15.1047, 2.486) (-15.0973, 2.4821) (-15.0899, 2.4782) (-15.0825, 2.4744) (-15.0752, 2.4706) (-15.0679, 2.4668) (-15.0606, 2.463) (-15.0533, 2.4593) (-15.0461, 2.4556) (-15.0388, 2.4519) (-15.0316, 2.4483) (-15.0245, 2.4447) (-15.0173, 2.4411) (-15.0102, 2.4375) (-15.0031, 2.434) (-14.996, 2.4305) (-14.9889, 2.427) (-14.9819, 2.4236) (-14.9749, 2.4201) (-14.9679, 2.4167) (-14.9609, 2.4134) (-14.954, 2.41) (-14.9471, 2.4067) (-14.9402, 2.4034) (-14.9334, 2.4002) (-14.9266, 2.397) (-14.9198, 2.3938) (-14.913, 2.3906) (-14.9062, 2.3874) (-14.8995, 2.3843) (-14.8928, 2.3812) (-14.8862, 2.3782) (-14.8795, 2.3751) (-14.8729, 2.3721) (-14.8663, 2.3691) (-14.8598, 2.3662) (-14.8533, 2.3633) (-14.8468, 2.3604) (-14.8403, 2.3575) (-14.8339, 2.3546) (-14.8275, 2.3518) (-14.8211, 2.349) (-14.8148, 2.3463) (-14.8084, 2.3435) (-14.8022, 2.3408) (-14.7959, 2.3381) (-14.7897, 2.3355) (-14.7835, 2.3328) (-14.7773, 2.3302) (-14.7712, 2.3277) (-14.7651, 2.3251) (-14.759, 2.3226) (-14.753, 2.3201) (-14.747, 2.3176) (-14.741, 2.3152) (-14.7351, 2.3128) (-14.7292, 2.3104) (-14.7233, 2.308) (-14.7175, 2.3057) (-14.7117, 2.3034) (-14.7059, 2.3011) (-14.7002, 2.2988) (-14.6945, 2.2966) (-14.6888, 2.2944) (-14.6832, 2.2922) (-14.6776, 2.29) (-14.672, 2.2879) (-14.6665, 2.2858) (-14.661, 2.2837) (-14.6556, 2.2817) (-14.6502, 2.2796) (-14.6448, 2.2776) (-14.6395, 2.2757) (-14.6342, 2.2737) (-14.6289, 2.2718) (-14.6237, 2.2699) (-14.6185, 2.268) (-14.6133, 2.2662) (-14.6082, 2.2644) (-14.6032, 2.2626) (-14.5981, 2.2608) (-14.5932, 2.259) (-14.5882, 2.2573) (-14.5833, 2.2556) (-14.5784, 2.2539) (-14.5736, 2.2523) (-14.5688, 2.2507) (-14.5641, 2.2491) (-14.5594, 2.2475) (-14.5547, 2.2459) (-14.5501, 2.2444) (-14.5455, 2.2429) (-14.541, 2.2414) (-14.5365, 2.24) (-14.5321, 2.2386) (-14.5277, 2.2372) (-14.5233, 2.2358) (-14.519, 2.2344) (-14.5147, 2.2331) (-14.5105, 2.2318) (-14.5063, 2.2305) (-14.5022, 2.2292) (-14.4981, 2.228) (-14.4941, 2.2268) (-14.4901, 2.2256) (-14.4862, 2.2244) (-14.4823, 2.2233) (-14.4785, 2.2222) (-14.4747, 2.2211) (-14.4709, 2.22) (-14.4673, 2.2189) (-14.4636, 2.2179) (-14.46, 2.2169) (-14.4565, 2.2159) (-14.453, 2.2149) (-14.4496, 2.214) (-14.4462, 2.2131) (-14.4429, 2.2122) (-14.4396, 2.2113) (-14.4364, 2.2104) (-14.4332, 2.2096) (-14.4301, 2.2088) (-14.427, 2.208) (-14.424, 2.2072) (-14.4211, 2.2065) (-14.4182, 2.2058) (-14.4154, 2.2051) (-14.4126, 2.2044) (-14.4099, 2.2037) (-14.4072, 2.2031) (-14.4046, 2.2025) (-14.4021, 2.2018) (-14.3996, 2.2013) (-14.3972, 2.2007) (-14.3948, 2.2002) (-14.3925, 2.1996) (-14.3903, 2.1991) (-14.3882, 2.1986) (-14.386, 2.1982) (-14.384, 2.1977) (-14.382, 2.1973) (-14.3801, 2.1969) (-14.3783, 2.1965) (-14.3765, 2.1961) (-14.3748, 2.1958) (-14.3732, 2.1954) (-14.3716, 2.1951) (-14.3701, 2.1948) (-14.3687, 2.1945) (-14.3673, 2.1943) (-14.366, 2.194) (-14.3648, 2.1938) (-14.3637, 2.1936) (-14.3626, 2.1934) (-14.3616, 2.1932) (-14.3607, 2.193) (-14.3598, 2.1929) (-14.3591, 2.1928) (-14.3584, 2.1926) (-14.3578, 2.1925) (-14.3572, 2.1924) (-14.3569, 2.1924) (-14.3566, 2.1923) (-14.3565, 2.1923) (-14.3564, 2.1923) knots -1 -1 -1 -1 -1 -1 -0.99583333 -0.99166667 -0.9875 -0.98333333 -0.97916667 -0.975 -0.97083333 -0.96666667 -0.9625 -0.95833333 -0.95416667 -0.95 -0.94583333 -0.94166667 -0.9375 -0.93333333 -0.92916667 -0.925 -0.92083333 -0.91666667 -0.9125 -0.90833333 -0.90416667 -0.9 -0.89583333 -0.89166667 -0.8875 -0.88333333 -0.87916667 -0.875 -0.87083333 -0.86666667 -0.8625 -0.85833333 -0.85416667 -0.85 -0.84583333 -0.84166667 -0.8375 -0.83333333 -0.82916667 -0.825 -0.82083333 -0.81666667 -0.8125 -0.80833333 -0.80416667 -0.8 -0.79583333 -0.79166667 -0.7875 -0.78333333 -0.77916667 -0.775 -0.77083333 -0.76666667 -0.7625 -0.75833333 -0.75416667 -0.75 -0.74583333 -0.74166667 -0.7375 -0.73333333 -0.72916667 -0.725 -0.72083333 -0.71666667 -0.7125 -0.70833333 -0.70416667 -0.7 -0.69583333 -0.69166667 -0.6875 -0.68333333 -0.67916667 -0.675 -0.67083333 -0.66666667 -0.6625 -0.65833333 -0.65416667 -0.65 -0.64583333 -0.64166667 -0.6375 -0.63333333 -0.62916667 -0.625 -0.62083333 -0.61666667 -0.6125 -0.60833333 -0.60416667 -0.6 -0.59583333 -0.59166667 -0.5875 -0.58333333 -0.57916667 -0.575 -0.57083333 -0.56666667 -0.5625 -0.55833333 -0.55416667 -0.55 -0.54583333 -0.54166667 -0.5375 -0.53333333 -0.52916667 -0.525 -0.52083333 -0.51666667 -0.5125 -0.50833333 -0.50416667 -0.5 -0.49583333 -0.49166667 -0.4875 -0.48333333 -0.47916667 -0.475 -0.47083333 -0.46666667 -0.4625 -0.45833333 -0.45416667 -0.45 -0.44583333 -0.44166667 -0.4375 -0.43333333 -0.42916667 -0.425 -0.42083333 -0.41666667 -0.4125 -0.40833333 -0.40416667 -0.4 -0.39583333 -0.39166667 -0.3875 -0.38333333 -0.37916667 -0.375 -0.37083333 -0.36666667 -0.3625 -0.35833333 -0.35416667 -0.35 -0.34583333 -0.34166667 -0.3375 -0.33333333 -0.32916667 -0.325 -0.32083333 -0.31666667 -0.3125 -0.30833333 -0.30416667 -0.3 -0.29583333 -0.29166667 -0.2875 -0.28333333 -0.27916667 -0.275 -0.27083333 -0.26666667 -0.2625 -0.25833333 -0.25416667 -0.25 -0.24583333 -0.24166667 -0.2375 -0.23333333 -0.22916667 -0.225 -0.22083333 -0.21666667 -0.2125 -0.20833333 -0.20416667 -0.2 -0.19583333 -0.19166667 -0.1875 -0.18333333 -0.17916667 -0.175 -0.17083333 -0.16666667 -0.1625 -0.15833333 -0.15416667 -0.15 -0.14583333 -0.14166667 -0.1375 -0.13333333 -0.12916667 -0.125 -0.12083333 -0.11666667 -0.1125 -0.10833333 -0.10416667 -0.1 -0.09583333 -0.09166667 -0.0875 -0.08333333 -0.07916667 -0.075 -0.07083333 -0.06666667 -0.0625 -0.05833333 -0.05416667 -0.05 -0.04583333 -0.04166667 -0.0375 -0.03333333 -0.02916667 -0.025 -0.02083333 -0.01666667 -0.0125 -0.00833333 -0.00416667 0 0 0 0 0 0
  line L118 (-14.3564, 2.1923) -> (-14.3558, 2.1922)
  line L119 (-14.3558, 2.1922) -> (-13.5924, 2.0756)
  circle A60 centre (0, 0) radius 10
  line L120 (0, 0) -> (0, -10)
  circle A61 centre (0, -10) radius 1.7
  circle A62 centre (7.0711, -7.0711) radius 1.7
  circle A63 centre (10, 0) radius 1.7
  circle A64 centre (7.0711, 7.0711) radius 1.7
  circle A65 centre (0, 10) radius 1.7
  circle A66 centre (-7.0711, 7.0711) radius 1.7
  circle A67 centre (-10, 0) radius 1.7
  circle A68 centre (-7.0711, -7.0711) radius 1.7
  dimension "d7" = 20
  dimension "d8" = 3.4
  dimension "d10" = 360
  constraint concentric A0 A60
  constraint coincident A0.centre A1.centre
  constraint coincident A60 L120.end
  constraint vertical L120
  constraint coincident L120.end A61.centre
  measures "d7" diameter of A60
  measures "d8" diameter of A61
extrude "押し出し3" cut sketch "スケッチ1 (2)" against normal blind 8 contours A60 A63 | A60 A63 | A60 A64 | A60 A64 | A60 A62 | A60 A62 | A60 A65 | A60 A65 | A60 A61 | A60 L120 A61 | A60 L120 A61 | A60 A66 | A60 A66 | A60 A68 | A60 A68 | A60 A67 | A60 A67 bodies 1 in component "Component"